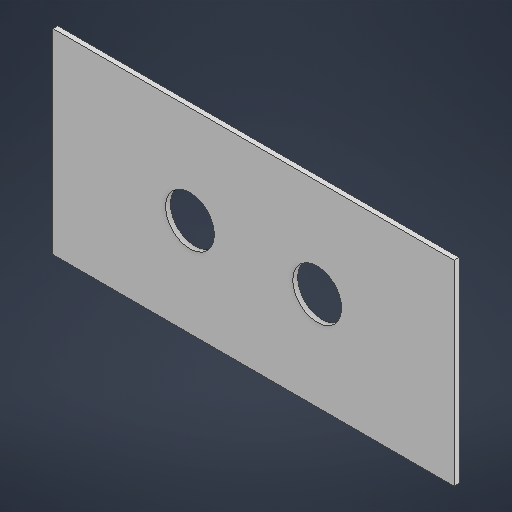
# Autodesk Inventor part: galvo spacer
Saved by Autodesk Inventor 2025 (Build 290162000, 162)
## iProperties
Created: 2024-07-17
Part Number: galvo spacer
Material: Generic
Document SubType Name: Modeling
Designer: mayhe
Density: 1 g/cm^3
Appearance: Default
Author: mayhe
Autodesk Inventor part; units mm, degrees
ref_plane "YZ Plane" through (0, 0, 0) normal (1, 0, 0) x (0, 1, 0)
ref_plane "XZ Plane" through (0, 0, 0) normal (0, 1, 0) x (-1, 0, 0)
ref_plane "XY Plane" through (0, 0, 0) normal (0, 0, 1) x (1, 0, 0)
sketch "Sketch1" plane through (0, 0, 0) normal (0, 0, 1) x (1, 0, 0)
  line L0 (-20.5, 10) -> (20.5, 10)
  line L1 (20.5, 10) -> (20.5, -10)
  line L2 (20.5, -10) -> (-20.5, -10)
  line L3 (-20.5, -10) -> (-20.5, 10)
  line L4 (-20.5, 10) -> (20.5, -10) construction
  line L5 (20.5, 10) -> (-20.5, -10) construction
  circle A0 centre (6.5, 0) radius 2.5
  circle A1 centre (-6.5, 0) radius 2.5
  point P0 (0, 0)
  dimension "d0" = 41
  dimension "d1" = 20
  dimension "d2" = 5
  dimension "d3" = 6.5
  dimension "d4" = 5
  dimension "d5" = 6.5
  constraints: 12 end point, 2 centre point, 2 midpoint, 2 parallel, 1 horizontal, 1 perpendicular
  measures "d0" distance of L1.end L2.end
  measures "d1" distance of L0.end L1.end
  measures "d2" diameter of A0
  measures "d3" distance of point (0, 0) A0.centre
  measures "d4" diameter of A1
  measures "d5" distance of point (0, 0) A1.centre
extrude "Extrusion1" add sketch "Sketch1" along normal mid plane 0.5
body "Solid1"
